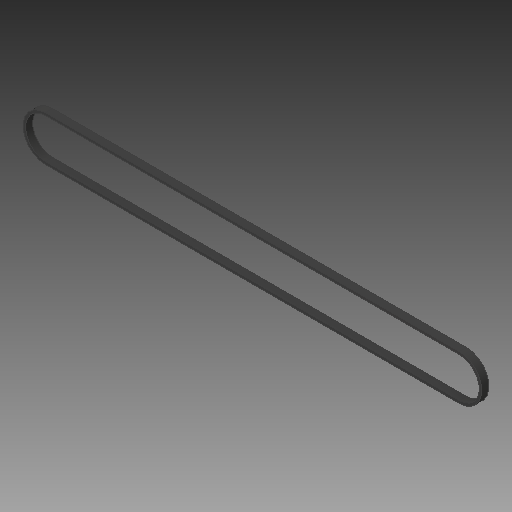
# Autodesk Inventor part: DGB_006_LonG Belt_Gates_1200-5M-09
Saved by Autodesk Inventor 2018.3 (Build 223284000, 284)
## iProperties
Created: 2020-01-18
Part Number: DGB_006_LonG Belt_Gates_1200-5M-09
Material: Generic
Document SubType Name: Modeling
Designer: myerpaul
Density: 1 g/cm^3
Appearance: Default
Mass: 34.4914 g
Surface Area: 293.917 cm^2
Volume: 34.4914 cm^3
Author: myerpaul
Autodesk Inventor part; units mm, degrees
ref_plane "YZ Plane" through (0, 0, 0) normal (1, 0, 0) x (0, 1, 0)
ref_plane "XZ Plane" through (0, 0, 0) normal (0, 1, 0) x (-1, 0, 0)
ref_plane "XY Plane" through (0, 0, 0) normal (0, 0, 1) x (1, 0, 0)
sketch "Sketch1" plane through (0, 0, 0) normal (0, 0, 1) x (1, 0, 0)
  circle A0 centre (0, 0) radius 24.892
  circle A1 centre (519.938, 0) radius 24.892
  line L0 (0, 0) -> (519.938, 0) construction
  line L1 (0, -25.019) -> (519.938, -25.019)
  line L2 (519.938, 25.019) -> (0, 25.019)
  arc A2 (0, 25.019) -> (0, -25.019) centre (0, 0) ccw
  arc A3 (519.938, -25.019) -> (519.938, 25.019) centre (519.938, 0) ccw
  line L3 (0, 28.194) -> (519.938, 28.194)
  arc A4 (519.938, -28.194) -> (519.938, 28.194) centre (519.938, 0) ccw
  line L4 (519.938, -28.194) -> (0, -28.194)
  arc A5 (0, 28.194) -> (0, -28.194) centre (0, 0) ccw
  line L5 (7.3323, 0) -> (3.6662, -6.35)
  line L6 (3.6662, -6.35) -> (-3.6662, -6.35)
  line L7 (-3.6662, -6.35) -> (-7.3323, 0)
  line L8 (-7.3323, 0) -> (-3.6662, 6.35)
  line L9 (-3.6662, 6.35) -> (3.6662, 6.35)
  line L10 (3.6662, 6.35) -> (7.3323, 0)
  line L11 (527.2703, 0) -> (523.6042, -6.35)
  line L12 (523.6042, -6.35) -> (516.2718, -6.35)
  line L13 (516.2718, -6.35) -> (512.6057, 0)
  line L14 (512.6057, 0) -> (516.2718, 6.35)
  line L15 (516.2718, 6.35) -> (523.6042, 6.35)
  line L16 (523.6042, 6.35) -> (527.2703, 0)
  point P0 (259.969, 0)
  dimension "d0" = 49.784
  dimension "d1" = 519.938
  dimension "d2" = 3.175
  dimension "d3" = 0.127
  dimension "d8" = 12.7
  constraints: 36 end point, 8 point on circle, 6 centre point, 4 tangent, 3 coincident, 2 parallel, 1 collinear, 1 equal radius, 1 horizontal, 1 horizontal alignment, 1 midpoint, 1 point on line, 29 other
  measures "d0" diameter of A0
  measures "d1" distance of L0.end point (0, 0)
  measures "d2" distance between parallel lines of L3 L2
  measures "d3" radial gap between concentric circles of A3 A1
  measures "d8" distance between parallel lines of L6 L9
extrude "Extrusion2" add sketch "Sketch1" along normal blind 9 contours L3 A4 L4 A5
body "Solid1"
body "Solid2"
